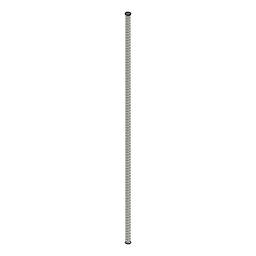
Сборка моя 2 шговых v1 (Autodesk Fusion 360 archive; units mm, degrees)
design "Направляющий винт"
Autodesk Fusion 360 part; units mm, degrees
sketch "Sketch1" plane through (0, 0, 0) normal (0, 0, 1) x (1, 0, 0)
  circle A0 centre (0, 0) radius 2.4955
  dimension "d1" = 4.991
  constraint coincident A0.centre origin
  measures "d1" diameter of A0
extrude "Extrude1" add sketch "Sketch1" along normal blind 250
thread "Thread1" "ISO Metric profile 5.0 M5x0.8 6g" major diameter 4.901 minor diameter 3.9895 pitch 0.8 angle 60 resizes the face on face at (-1.5192, 1.9798, 166.6667)

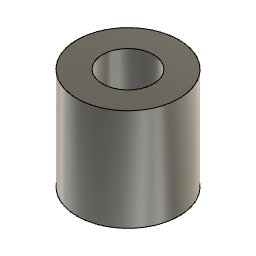
design "Муфта"
Autodesk Fusion 360 part; units mm, degrees
sketch "Sketch1" plane through (0, 0, 0) normal (0, 0, 1) x (1, 0, 0)
  circle A0 centre (10, 10) radius 2.4955
  circle A1 centre (10, 10) radius 5
  dimension "d1" = 4.991
  dimension "d2" = 10
  constraint concentric A0 A1
  measures "d1" diameter of A0
  measures "d2" diameter of A1
extrude "Extrude1" add sketch "Sketch1" along normal blind 10

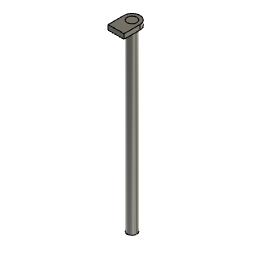
design "Вал"
Autodesk Fusion 360 part; units mm, degrees
sketch "Sketch1" plane through (0, 0, 0) normal (0, 0, 1) x (1, 0, 0)
  circle A0 centre (0, 0) radius 3
  dimension "d1" = 6
  constraint coincident A0.centre origin
  measures "d1" diameter of A0
extrude "Extrude1" add sketch "Sketch1" along normal blind 115 makes body 1
sketch "Sketch2" plane through (0, 0, 0) normal (0, 0, 1) x (1, 0, 0)
  circle A0 centre (15, 25) radius 3
  circle A1 centre (15, 25) radius 5
  dimension "d4" = 6
  dimension "d5" = 10
  constraint concentric A0 A1
  measures "d4" diameter of A0
  measures "d5" diameter of A1
extrude "Extrude2" add sketch "Sketch2" along normal blind 3 separate body makes body 2
sketch "Sketch4" plane through (0, 0, 0) normal (0, 0, 1) x (1, 0, 0)
  line L0 (10, 25) -> (10, 15)
  line L1 (10, 15) -> (20, 15)
  line L2 (20, 15) -> (20, 25)
  line L3 (10, 25) -> (20, 25)
  constraint vertical L0
  constraint perpendicular L0 L1
  constraint perpendicular L1 L2
  constraint perpendicular L2 L3
extrude "Extrude3" add sketch "Sketch4" along normal blind 3 bodies 2
sketch "Sketch5" plane through (0, 0, 3) normal (0, 0, 1) x (-1, 0, 0)
  arc A0 (-18, -25) -> (-12, -25) centre (-15, -25) ccw
  line L0 (-18, -25) -> (-12, -25)
  arc A1 (-20, -25) -> (-10, -25) centre (-15, -25) ccw
  line L1 (-10, -25) -> (-10, -15)
  line L2 (-10, -15) -> (-20, -15)
  line L3 (-20, -15) -> (-20, -25)
  circle A2 centre (-15, -25) radius 3
  constraint concentric A0 A2
extrude "Extrude4" cut sketch "Sketch5" against normal blind 13 contours L0 A2 bodies 2
move_body "Align1" bodies 2 to x (1, 0, 0) y (0, 1, 0) z (0, 0, 1) at (-15, -25, 112)

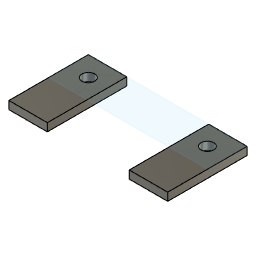
design "Каретка"
Autodesk Fusion 360 part; units mm, degrees
sketch "Sketch1" plane through (0, 0, 0) normal (0, 0, 1) x (1, 0, 0)
  line L0 (0, 0) -> (200, 0)
  line L1 (200, 0) -> (200, 50)
  line L2 (200, 50) -> (0, 50)
  line L3 (0, 50) -> (0, 0)
  dimension "d1" = 200
  dimension "d2" = 50
  constraint horizontal L0
  constraint vertical L1
  constraint horizontal L2
  constraint vertical L3
  constraint coincident L0.start L3.end
  measures "d1" distance of L0.start L0.end
  measures "d2" distance of L0.start L2.end
extrude "Extrude1" add sketch "Sketch1" along normal blind 10 makes body 1
sketch "Sketch2" plane through (0, 0, 10) normal (0, 0, 1) x (-1, 0, 0)
  line L0 (0, -50) -> (0, 0)
  line L1 (0, 0) -> (-200, 0)
  line L2 (-200, 0) -> (-200, -50)
  line L3 (-200, -50) -> (0, -50)
sketch "Sketch3" plane through (0, 0, 10) normal (0, 0, 1) x (-1, 0, 0)
  circle A0 centre (-175, -25) radius 8
  circle A1 centre (-25, -25) radius 8
  dimension "d9" = 16
  dimension "d10" = 16
  measures "d9" diameter of A0
  measures "d10" diameter of A1
extrude "Extrude2" cut sketch "Sketch3" against normal blind 90 bodies 1
sketch "Sketch4" plane through (0, 0, 10) normal (0, 0, 1) x (-1, 0, 0)
  circle A0 centre (-100, -25) radius 2.4955
  dimension "d14" = 4.991
  measures "d14" diameter of A0
extrude "Extrude3" cut sketch "Sketch4" against normal blind 55 bodies 1
extrude "Extrude4" add 1 faces at (66.6667, 0, 3.3333) along direction (0, -1, 0) blind 50 on bodies 1 bodies 1
sketch "Sketch5" plane through (0, 0, 10) normal (0, 0, 1) x (-1, 0, 0)
  circle A0 centre (-100, -25) radius 2.4955
  circle A1 centre (-25, -25) radius 8
  circle A2 centre (-175, -25) radius 8
  line L0 (0, -50) -> (0, 50)
  line L1 (0, 50) -> (-200, 50)
  line L2 (-200, 50) -> (-200, -50)
  line L3 (-200, -50) -> (0, -50)
  line L4 (0, -50) -> (-200, 50) construction
  line L5 (-200, -50) -> (0, 50) construction
  line L6 (-100, 0) -> (-100, -50) construction
  line L7 (-48.4203, 50) -> (-151.5797, 50)
  line L8 (-151.5797, 50) -> (-151.5797, -50)
  line L9 (-151.5797, -50) -> (-48.4203, -50)
  line L10 (-48.4203, -50) -> (-48.4203, 50)
  line L11 (-48.4203, 50) -> (-151.5797, -50) construction
  line L12 (-151.5797, 50) -> (-48.4203, -50) construction
  point P0 (-100, 0)
  constraint coincident L0.start L3.end
  constraint coincident L1.end L2.start
  constraint coincident L2.end L3.start
  constraint coincident L0.end L1.start
  constraint midpoint L4 P0
  constraint midpoint L3 L6.end
  constraint horizontal L7
  constraint perpendicular L7 L8
  constraint parallel L7 L9
  constraint parallel L8 L10
  constraint coincident L1 L7.start
  constraint coincident L11 P0
  constraint coincident L12 P0
  constraint coincident P0 L6.start
extrude "Extrude5" cut sketch "Sketch5" against normal blind 55 contours L1 L3 L7 L8 L9 L10 bodies 1 makes body 2 at (24.2742, -27.6592, 10)

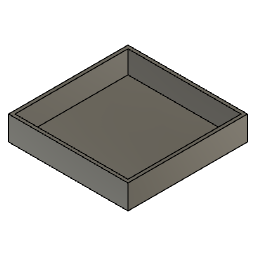
design "Ванна"
Autodesk Fusion 360 part; units mm, degrees
sketch "Sketch1" plane through (0, 0, 0) normal (0, 0, 1) x (1, 0, 0)
  line L0 (0, 0) -> (350, 0)
  line L1 (350, 0) -> (350, 350)
  line L2 (350, 350) -> (0, 350)
  line L3 (0, 350) -> (0, 0)
  line L4 (-10, 0) -> (-10, -10)
  line L5 (-10, -10) -> (360, -10)
  line L6 (360, -10) -> (360, 360)
  line L7 (360, 360) -> (-10, 360)
  line L8 (-10, 360) -> (-10, -10)
  dimension "d1" = 350
  dimension "d2" = 350
  dimension "d3" = 10
  dimension "d4" = 370
  dimension "d5" = 370
  constraint horizontal L0
  constraint vertical L1
  constraint horizontal L2
  constraint vertical L3
  constraint coincident L0.start L3.end
  constraint horizontal L5
  constraint vertical L6
  constraint horizontal L7
  constraint vertical L8
  measures "d1" distance of L0.start L0.end
  measures "d2" distance of L0.start L2.end
  measures "d3" distance of L0.start L4.start
  measures "d4" distance of L4.end L5.end
  measures "d5" distance of L4.end L7.end
extrude "Extrude1" add sketch "Sketch1" along normal blind 75
sketch "Sketch2" plane through (0, 0, 0) normal (0, 0, 1) x (1, 0, 0)
  line L0 (0, 350) -> (350, 350)
  line L1 (350, 350) -> (350, 0)
  line L2 (350, 0) -> (0, 0)
  line L3 (0, 0) -> (0, 350)
  constraint horizontal L0
  constraint vertical L1
  constraint horizontal L2
  constraint vertical L3
extrude "Extrude2" add sketch "Sketch2" along normal blind 5

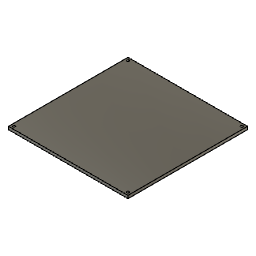
design "Платформа"
Autodesk Fusion 360 part; units mm, degrees
sketch "Sketch1" plane through (0, 0, 0) normal (0, 0, 1) x (1, 0, 0)
  line L0 (0, 0) -> (420, 0)
  line L1 (420, 0) -> (420, 420)
  line L2 (420, 420) -> (0, 420)
  line L3 (0, 420) -> (0, 0)
  dimension "d1" = 420
  dimension "d2" = 420
  constraint horizontal L0
  constraint vertical L1
  constraint horizontal L2
  constraint vertical L3
  constraint coincident L0.start L3.end
  measures "d1" distance of L0.start L0.end
  measures "d2" distance of L0.start L2.end
extrude "Extrude1" add sketch "Sketch1" along normal blind 20
sketch "Sketch2" plane through (0, 0, 20) normal (0, 0, 1) x (-1, 0, 0)
  line L0 (0, -420) -> (0, 0)
  line L1 (0, 0) -> (-420, 0)
  line L2 (-420, 0) -> (-420, -420)
  line L3 (-420, -420) -> (0, -420)
  circle A0 centre (-410, -410) radius 4
  circle A1 centre (-10, -410) radius 4
  circle A2 centre (-410, -10) radius 4
  circle A3 centre (-10, -10) radius 4
  dimension "d7" = 400
  dimension "d8" = 8
  dimension "d9" = 8
  dimension "d10" = 400
  dimension "d11" = 400
  dimension "d12" = 8
  dimension "d13" = 8
  measures "d7" distance of A0.centre A1.centre
  measures "d8" diameter of A0
  measures "d9" diameter of A1
  measures "d10" distance of A1.centre A3.centre
  measures "d11" distance of A0.centre A2.centre
  measures "d12" diameter of A2
  measures "d13" diameter of A3
extrude "Extrude2" cut sketch "Sketch2" against normal blind 100 contours A0 | A1 | A2 | A3
extrude "Extrude3" cut 1 faces at (144.2065, 144.341, 20) along direction (0, 0, -1) blind 10

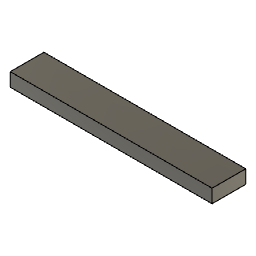
design "Платформа для двигателя"
Autodesk Fusion 360 part; units mm, degrees
sketch "Sketch1" plane through (0, 0, 0) normal (0, 0, 1) x (1, 0, 0)
  line L0 (10, 10) -> (310, 10)
  line L1 (310, 10) -> (310, 60)
  line L2 (310, 60) -> (10, 60)
  line L3 (10, 60) -> (10, 10)
  dimension "d1" = 300
  dimension "d2" = 50
  constraint horizontal L0
  constraint vertical L1
  constraint horizontal L2
  constraint vertical L3
  measures "d1" distance of L0.start L0.end
  measures "d2" distance of L0.start L2.end
extrude "Extrude1" add sketch "Sketch1" along normal blind 20
